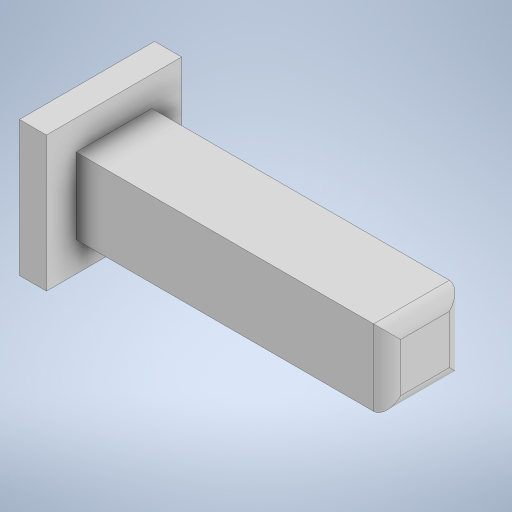
# Autodesk Inventor part: Enclosure_Button
Saved by Autodesk Inventor 2023 (Build 270158030, 158C)
## iProperties
Created: 2024-02-03
Part Number: Enclosure_Button
Material: Generic
Document SubType Name: Modeling
Designer: Fabian
Density: 1 g/cm^3
Appearance: Default
Author: Fabian
Autodesk Inventor part; units mm, degrees
ref_plane "YZ Plane" through (0, 0, 0) normal (1, 0, 0) x (0, 1, 0)
ref_plane "XZ Plane" through (0, 0, 0) normal (0, 1, 0) x (-1, 0, 0)
ref_plane "XY Plane" through (0, 0, 0) normal (0, 0, 1) x (1, 0, 0)
sketch "Sketch1" plane through (0, 0, 0) normal (1, 0, 0) x (0, 1, 0)
  line L0 (7.7173, 6.935) -> (2.7173, 6.935)
  line L1 (2.7173, 6.935) -> (2.7173, 1.935)
  line L2 (2.7173, 1.935) -> (7.7173, 1.935)
  line L3 (7.7173, 1.935) -> (7.7173, 6.935)
  point P0 (0, 0)
  dimension "d0" = 5
  dimension "d1" = 5
  constraints: 8 end point, 2 parallel, 1 horizontal, 1 perpendicular
  measures "d0" distance of L2.end L1.end
  measures "d1" distance of L1.end L0.end
extrude "Extrusion1" add sketch "Sketch1" along normal blind 1
sketch "Sketch2" plane through (1, 0, 0) normal (1, 0, 0) x (0, 0, -1)
  line L0 (-5.835, 6.6173) -> (-3.035, 6.6173)
  line L1 (-3.035, 6.6173) -> (-3.035, 3.8173)
  line L2 (-3.035, 3.8173) -> (-5.835, 3.8173)
  line L3 (-5.835, 3.8173) -> (-5.835, 6.6173)
  line L4 (-1.935, 7.7173) -> (-6.935, 7.7173) projected
  line L5 (-6.935, 7.7173) -> (-6.935, 2.7173) projected
  point P0 (0, 0)
  point P1 (-5.835, 5.2173)
  point P2 (-6.935, 5.2173)
  dimension "d4" = 2.8
  dimension "d5" = 2.8
  dimension "d6" = 1.1
  dimension "d7" = 1.1
  constraints: 8 end point, 2 midpoint, 2 parallel, 1 horizontal, 1 perpendicular
  measures "d4" distance of L1.end L2.end
  measures "d5" distance of L0.end L1.end
  measures "d6" distance between parallel lines of L4 L0
  measures "d7" distance of point (-5.835, 5.217) point (-6.935, 5.217)
extrude "Extrusion2" add sketch "Sketch2" along normal blind 11.5
fillet "Fillet1" radius 0.5 4 edges at (12.5, 5.2173, 5.835) (12.5, 6.6173, 4.435) (12.5, 5.2173, 3.035) (12.5, 3.8173, 4.435)
body "Solid1"
